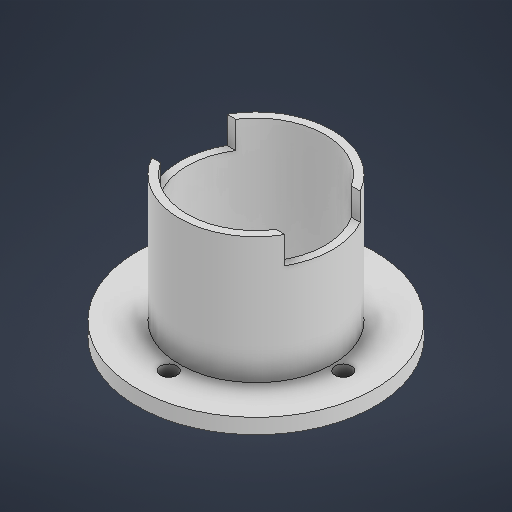
# Autodesk Inventor part: PZT holder
Saved by Autodesk Inventor 2025 (Build 290162000, 162)
## iProperties
Created: 2024-09-30
Part Number: PZT holder
Material: Generic
Document SubType Name: Modeling
Designer: mayhe
Density: 1 g/cm^3
Appearance: Default
Author: mayhe
Autodesk Inventor part; units mm, degrees
ref_plane "YZ Plane" through (0, 0, 0) normal (1, 0, 0) x (0, 1, 0)
ref_plane "XZ Plane" through (0, 0, 0) normal (0, 1, 0) x (-1, 0, 0)
ref_plane "XY Plane" through (0, 0, 0) normal (0, 0, 1) x (1, 0, 0)
sketch "Sketch1" plane through (0, 0, 0) normal (0, 1, 0) x (-1, 0, 0)
  circle A0 centre (0, 0) radius 22.9
  circle A1 centre (0, 0) radius 39.5
  circle A2 centre (0, 0) radius 29
  circle A3 centre (0, -29) radius 2.75
  circle A4 centre (29, 0) radius 2.75
  circle A5 centre (0, 29) radius 2.75
  circle A6 centre (-29, 0) radius 2.75
  circle A7 centre (0, 0) radius 25.4
  line L0 (-29, 12.5) -> (29, 12.5)
  line L1 (29, 12.5) -> (29, -12.5)
  line L2 (29, -12.5) -> (-29, -12.5)
  line L3 (-29, -12.5) -> (-29, 12.5)
  line L4 (-29, 12.5) -> (29, -12.5) construction
  line L5 (29, 12.5) -> (-29, -12.5) construction
  point P0 (19.1875, 12.5)
  point P1 (22.1113, 12.5)
  point P2 (-22.1113, 12.5)
  point P3 (-19.1875, 12.5)
  point P4 (-19.1875, -12.5)
  point P5 (-22.1113, -12.5)
  point P6 (22.1113, -12.5)
  point P7 (19.1875, -12.5)
  dimension "d2" = 58
  dimension "d0" = 45.8
  dimension "d1" = 79
  dimension "d3" = 5.5
  dimension "d6" = 360
  dimension "d10" = 25
  constraints: 12 end point, 7 centre point, 4 coincident, 2 midpoint, 2 parallel, 1 horizontal, 1 perpendicular, 1 vertical alignment, 11 other
  measures "d0" diameter of A0
  measures "d1" diameter of A1
  measures "d3" diameter of A3
  measures "d10" distance of L0.end L1.end
extrude "Extrusion1" add sketch "Sketch1" along normal blind 5 contours A0 L2 L0 | A0 L0 A7 L2 | L0 A0 | A0 L0 A7 | L2 A7 A0 | A0 L2 | A0 L2 A7 L0 | L0 A2 A4 L2 A7 | A7 L0 A2 A5 | L2 A2 A3 A7 | A7 L2 A2 A6 L0 | L0 L1 A4 A2 | A2 A4 L1 L2 | A2 A6 L3 L0 | L2 L3 A6 A2 | A1
extrude "Extrusion2" add sketch "Sketch1" along normal blind 47 contours A0 L0 A7 | L2 A7 A0
extrude "Extrusion3" add sketch "Sketch1" along normal blind 38 contours A0 L0 A7 L2 | A0 L2 A7 L0
body "Solid1"
